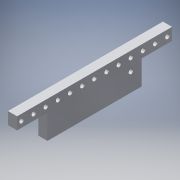
# Autodesk Inventor part: SpanRearAndMiddleSupport
Saved by Autodesk Inventor 2016 SP1 (Build 200210100, 210)
## iProperties
Created: 2016-02-14
Part Number: SpanRearAndMiddleSupport
Material: Aluminum 6061
Document SubType Name: Modeling
Designer: steele
Density: 2.7 g/cm^3
Appearance: Aluminum - Flat
Mass: 628.65 g
Surface Area: 453.434 cm^2
Volume: 232.833 cm^3
Author: steele
Autodesk Inventor part; units mm, degrees
ref_plane "YZ Plane" through (0, 0, 0) normal (1, 0, 0) x (0, 1, 0)
ref_plane "XZ Plane" through (0, 0, 0) normal (0, 1, 0) x (-1, 0, 0)
ref_plane "XY Plane" through (0, 0, 0) normal (0, 0, 1) x (1, 0, 0)
sketch "Sketch2" plane through (0, 0, 0) normal (1, 0, 0) x (0, 1, 0)
  line L0 (0, 0) -> (0, 95.25)
  line L1 (0, 95.25) -> (50.8, 95.25)
  line L2 (50.8, 95.25) -> (50.8, 158.75)
  line L3 (50.8, 158.75) -> (76.2, 158.75)
  line L4 (76.2, 158.75) -> (76.2, 15.0657)
  line L5 (76.2, 15.0657) -> (76.2, 0)
  line L6 (76.2, 0) -> (0, 0) construction
  line L7 (0, 0) -> (0, -95.25)
  line L8 (0, -95.25) -> (50.8, -95.25)
  line L9 (50.8, -95.25) -> (50.8, -158.75)
  line L10 (50.8, -158.75) -> (76.2, -158.75)
  line L11 (76.2, -158.75) -> (76.2, -15.0657)
  line L12 (76.2, -15.0657) -> (76.2, 0)
  dimension "d5" = 50.8
  dimension "d6" = 25.4
  dimension "d8" = 63.5
  dimension "d9" = 95.25
  constraints: 26 end point, 5 symmetric about line, 3 perpendicular, 3 vertical, 1 horizontal
  measures "d5" distance of L0.end L1.end
  measures "d6" distance of L2.end L3.end
  measures "d8" distance of L1.end L2.end
  measures "d9" distance of L0.start L0.end
extrude "Extrusion1" add sketch "Sketch2" along normal mid plane 19.05
sketch "Sketch3" plane through (9.525, 50.8, -95.25) normal (0, 0, -1) x (-1, 0, 0)
  line L0 (19.05, 0) -> (19.05, 25.4) projected
  line L1 (0, -50.8) -> (19.05, -50.8)
  line L2 (19.05, -50.8) -> (19.05, 0)
  line L3 (19.05, 0) -> (0, 0)
  line L4 (0, 0) -> (0, -50.8)
  point P0 (9.525, -50.8)
  constraints: 8 end point, 2 parallel, 1 horizontal, 1 perpendicular
extrude "Extrusion2" add sketch "Sketch3" along normal blind 6.35
sketch "Sketch4" plane through (9.525, 76.2, -158.75) normal (0, 0, -1) x (-1, 0, 0)
  line L0 (0, 0) -> (0, -25.4) projected
  line L1 (19.05, -25.4) -> (19.05, 0) projected
  line L2 (0, 0) -> (19.05, 0)
  line L3 (19.05, 0) -> (19.05, -25.4)
  line L4 (19.05, -25.4) -> (0, -25.4)
  line L5 (0, -25.4) -> (0, 0)
  point P0 (9.525, -76.2)
  constraints: 8 end point, 2 parallel, 1 horizontal, 1 perpendicular
extrude "Extrusion3" add sketch "Sketch4" along normal blind 6.35
sketch "Sketch5" plane through (9.525, 0, 0) normal (1, 0, 0) x (0, 0, -1)
  line L0 (-158.75, 76.2) -> (-158.75, 50.8) construction
  line L1 (-158.75, 63.5) -> (113.5145, 63.5) construction
  circle A0 centre (-149.225, 63.5) radius 4.7625
  circle A1 centre (-123.825, 63.5) radius 4.7625
  circle A2 centre (-98.425, 63.5) radius 4.7625
  circle A3 centre (-73.025, 63.5) radius 4.7625
  circle A4 centre (-47.625, 63.5) radius 4.7625
  circle A5 centre (-22.225, 63.5) radius 4.7625
  circle A6 centre (3.175, 63.5) radius 4.7625
  circle A7 centre (28.575, 63.5) radius 4.7625
  circle A8 centre (53.975, 63.5) radius 4.7625
  circle A9 centre (79.375, 63.5) radius 4.7625
  circle A10 centre (104.775, 63.5) radius 4.7625
  circle A11 centre (130.175, 63.5) radius 4.7625
  circle A12 centre (155.575, 63.5) radius 4.7625
  point P0 (0, 0)
  dimension "d16" = 9.525
  dimension "d17" = 9.525
  dimension "d20" = 25.4
  constraints: 13 centre point, 2 end point, 2 horizontal, 1 midpoint, 1 point on line, 24 other
  measures "d16" diameter of A0
  measures "d17" distance from line of A0.centre L0
  measures "d20" distance of A0.centre A1.centre
extrude "Extrusion4" cut sketch "Sketch5" against normal through all
sketch "Sketch6" plane through (9.525, 0, 0) normal (1, 0, 0) x (0, 0, -1)
  line L0 (-95.25, 50.8) -> (-95.25, 0) construction
  line L1 (-95.25, 38.1) -> (101.6, 38.1) construction
  line L2 (101.6, 50.8) -> (101.6, 0) construction
  line L3 (-158.75, 76.2) -> (165.1, 76.2) construction
  circle A0 centre (79.375, 38.1) radius 4.7625
  line L4 (165.1, 76.2) -> (165.1, 50.8) projected
  point P0 (0, 0)
  dimension "d28" = 38.1
  dimension "d29" = 85.725
  dimension "d30" = 9.525
  constraints: 3 point on line, 2 end point, 1 centre point, 1 horizontal
  measures "d28" distance between parallel lines of L1 L3
  measures "d29" distance from line of A0.centre L4
  measures "d30" diameter of A0
extrude "Extrusion5" cut sketch "Sketch6" against normal through all
body "Solid1"
